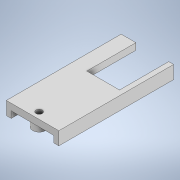
# Autodesk Inventor part: power_halterung
Saved by Autodesk Inventor 2021 (Build 250183000, 183)
## iProperties
Created: 2021-08-30
Part Number: power_halterung
Material: Generisch
Document SubType Name: Modeling
Designer: Tilman
Density: 1 g/cm^3
Appearance: Vorgabe
Author: Tilman
Autodesk Inventor part; units mm, degrees
ref_plane "YZ Plane" through (0, 0, 0) normal (1, 0, 0) x (0, 1, 0)
ref_plane "XZ Plane" through (0, 0, 0) normal (0, 1, 0) x (-1, 0, 0)
ref_plane "XY Plane" through (0, 0, 0) normal (0, 0, 1) x (1, 0, 0)
sketch "Skizze1" plane through (0, 0, 0) normal (0, 1, 0) x (-1, 0, 0)
  line L0 (0, 0) -> (0, -35)
  line L1 (0, -35) -> (-4.5, -35)
  line L2 (-4.5, -35) -> (-4.5, -20)
  line L3 (-4.5, -20) -> (-14.5, -20)
  line L4 (-14.5, -20) -> (-14.5, -35)
  line L5 (-14.5, -35) -> (-16, -35)
  line L6 (-16, -35) -> (-16, 0)
  line L7 (-16, 0) -> (0, 0)
  circle A0 centre (-8, -2) radius 0.95
  point P0 (-8, 0)
  dimension "d0" = 16
  dimension "d1" = 1.9
  dimension "d2" = 2
  dimension "d4" = 33
  dimension "d5" = 15
  dimension "d6" = 10
  dimension "d7" = 4.5
  constraints: 16 end point, 6 perpendicular, 2 point on line, 1 centre point, 1 midpoint, 1 vertical, 1 vertical alignment
  measures "d0" distance of L6.end L0.start
  measures "d1" diameter of A0
  measures "d2" distance from line of L7 A0.centre
  measures "d4" distance from line of A0.centre L5
  measures "d5" distance of L1.end L2.end
  measures "d6" distance of L2.end L3.end
  measures "d7" distance of L0.end L1.end
extrude "Extrusion1" add sketch "Skizze1" against normal blind 2
sketch "Skizze2" plane through (0, -2, 0) normal (0, -1, 0) x (1, 0, 0)
  line L0 (16, -35) -> (16, 0) projected
  line L1 (16, 0) -> (0, 0) projected
  line L2 (0, 0) -> (0, -35) projected
  line L3 (0, -35) -> (4.5, -35) projected
  line L4 (4.5, -35) -> (4.5, -20) projected
  line L5 (4.5, -20) -> (14.5, -20) projected
  line L6 (14.5, -20) -> (14.5, -35) projected
  line L7 (14.5, -35) -> (16, -35) projected
  circle A0 centre (8, -2) radius 0.95 projected
  circle A1 centre (8, -2) radius 1.95
  line L8 (0, 0) -> (16, 0) projected
  line L9 (1.5, 0) -> (1.5, -35)
  line L10 (0, -35) -> (4.5, -35) projected
  line L11 (14.5, -35) -> (16, -35) projected
  line L12 (14.5, -20) -> (14.5, 0)
  point P0 (14.5, 0)
  dimension "d10" = 1
  dimension "d11" = 1.5
  constraints: 4 end point, 3 point on line, 2 vertical, 1 centre point
  measures "d10" radial gap between concentric circles of A0 A1
  measures "d11" distance between parallel lines of L2 L9
extrude "Extrusion2" add sketch "Skizze2" along normal blind 2 contours L7 L6 L12 L1 L0 | L9 L3 L2 L1 | A1
